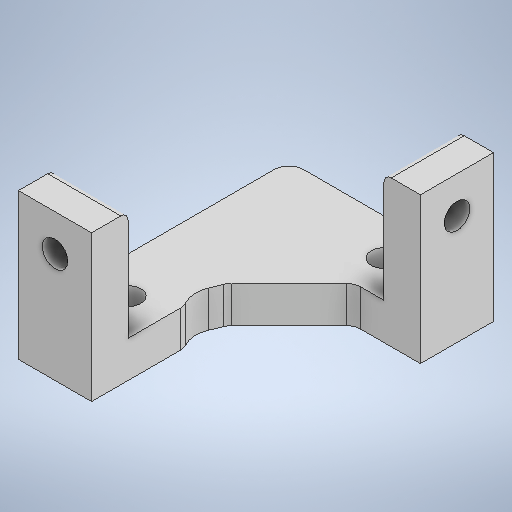
# Autodesk Inventor part: B8-FR-case-bracket
Saved by Autodesk Inventor 2025.2 (Build 292293000, 293)
## iProperties
Created: 2025-11-15
Part Number: B8-FR-case-bracket
Material: 일반
Document SubType Name: Modeling
Designer: RunGeun
Density: 1 g/cm^3
Appearance: 기본값
Author: RunGeun
Autodesk Inventor part; units mm, degrees
ref_plane "YZ Plane" through (0, 0, 0) normal (1, 0, 0) x (0, 1, 0)
ref_plane "XZ Plane" through (0, 0, 0) normal (0, 1, 0) x (-1, 0, 0)
ref_plane "XY Plane" through (0, 0, 0) normal (0, 0, 1) x (1, 0, 0)
sketch "스케치1" plane through (0, 0, 0) normal (0, 1, 0) x (-1, 0, 0)
  circle A0 centre (5.2143, -44.8531) radius 1.75
  circle A1 centre (18.2143, -22.8531) radius 1.75
  line L0 (23.2143, -12.8531) -> (13.2143, -12.8531)
  line L1 (-4.7857, -39.8531) -> (-4.7857, -49.8531)
  line L2 (-4.7857, -49.8531) -> (23.2143, -49.8531)
  line L3 (23.2143, -49.8531) -> (23.2143, -12.8531)
  line L4 (13.2143, -39.8531) -> (-4.7857, -39.8531)
  circle A2 centre (10.2143, -27.8531) radius 3.75
  line L5 (13.2143, -12.8531) -> (13.2143, -25.6031)
  line L6 (13.2143, -30.1031) -> (13.2143, -39.8531)
  line L7 (-4.7857, -49.8531) -> (0.2143, -49.8531)
  line L8 (0.2143, -49.8531) -> (0.2143, -39.8531)
  line L9 (0.2143, -39.8531) -> (-4.7857, -39.8531)
  line L10 (-4.7857, -39.8531) -> (-4.7857, -49.8531)
  line L11 (13.2143, -12.8531) -> (23.2143, -12.8531)
  line L12 (23.2143, -12.8531) -> (23.2143, -17.8531)
  line L13 (23.2143, -17.8531) -> (13.2143, -17.8531)
  line L14 (13.2143, -17.8531) -> (13.2143, -12.8531)
  point P0 (0, 0)
  dimension "d0" = 22
  dimension "d1" = 13
  dimension "d2" = 3.5
  dimension "d3" = 3.5
  dimension "d5" = 5
  dimension "d6" = 10
  dimension "d7" = 10
  dimension "d8" = 5
  dimension "d9" = 5
  dimension "d10" = 7.5
  dimension "d13" = 5
  dimension "d15" = 8
  dimension "d16" = 10
  dimension "d17" = 0
  dimension "d18" = 5
  dimension "d19" = 5
  dimension "d20" = 5
  constraints: 30 end point, 6 parallel, 3 centre point, 3 horizontal, 3 perpendicular, 2 point on circle, 2 point on line
  measures "d0" vertical distance of A1.centre A0.centre
  measures "d1" horizontal distance of A0.centre A1.centre
  measures "d2" diameter of A0
  measures "d3" diameter of A1
  measures "d5" distance from line of A1.centre L3
  measures "d6" distance from line of A1.centre L0
  measures "d7" distance from line of A0.centre L1
  measures "d8" distance from line of A0.centre L4
  measures "d9" distance from line of A0.centre L2
  measures "d10" diameter of A2
  measures "d13" distance from line of A1.centre L5
  measures "d15" horizontal distance of A1.centre A2.centre
  measures "d16" distance of L0.start L0.end
  measures "d17" distance between parallel lines of L5 L6
  measures "d18" vertical distance of A2.centre A1.centre
  measures "d19" distance of L9.end L8.end
  measures "d20" distance of L11.end L12.end
extrude "돌출1" add sketch "스케치1" along normal blind 5 contours L3 L2 L8 L4 L6 A2 L5 L13
extrude "돌출2" add sketch "스케치1" along normal blind 20 contours L3 L13 L5 L0 | L2 L1 L4 L8
sketch "스케치2" plane through (-0.2143, 5, -39.8531) normal (-1, 0, 0) x (0, 0, 1)
  circle A0 centre (-5, 10) radius 1.75
  line L0 (0, 0) -> (0, 15) projected
  line L1 (-10, 15) -> (0, 15) projected
  point P0 (39.8531, -5)
  dimension "d25" = 3.5
  dimension "d26" = 5
  dimension "d27" = 5
  constraints: 1 centre point
  measures "d25" diameter of A0
  measures "d26" distance from line of A0.centre L0
  measures "d27" distance from line of L1 A0.centre
extrude "돌출3" cut sketch "스케치2" against normal blind 20
sketch "스케치3" plane through (-13.2143, 5, -17.8531) normal (0, 0, -1) x (-1, 0, 0)
  circle A0 centre (5, 10) radius 1.75
  line L0 (0, 15) -> (10, 15) projected
  line L1 (10, 0) -> (10, 15) projected
  point P0 (-13.2143, -5)
  dimension "d30" = 3.5
  dimension "d31" = 5
  dimension "d32" = 5
  constraints: 1 centre point
  measures "d30" diameter of A0
  measures "d31" distance from line of A0.centre L0
  measures "d32" distance from line of L1 A0.centre
extrude "돌출4" cut sketch "스케치3" against normal blind 20
chamfer "모따기1" distance 9 angle 45 1 edges at (-13.2143, 2.5, -39.8531)
fillet "모깎기1" radius 2 4 edges at (-13.2143, 2.5, -30.8531) (-4.2143, 2.5, -39.8531) (-23.2143, 2.5, -49.8531) (-13.2143, 2.5, -25.6031)
fillet "모깎기2" radius 80 1 edges at (-13.2127, 2.5, -30.1052)
fillet "모깎기3" radius 1 2 edges at (-0.2143, 20, -44.8531) (-18.2143, 20, -17.8531)
equation "\"d3\" = d2"
equation "\"d7\" = d6"
equation "\"d8\" = d5"
equation "\"d9\" = d5"
equation "\"d13\" = d5"
equation "\"d20\" = d19"
equation "\"d27\" = d26"
equation "\"d32\" = d31"
equation "\"d4\" = d5"
